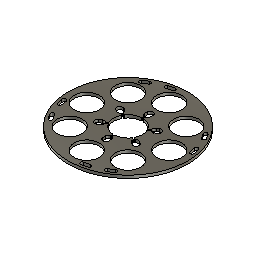
Laser Cut Spool (Autodesk Fusion 360 design; units mm, degrees)
Autodesk Fusion 360 part; units mm, degrees
sketch "Sketch1" plane through (0, 0, 0) normal (0, 0, 1) x (1, 0, 0)
  circle A0 centre (0, 0) radius 100
  circle A1 centre (0, 0) radius 38
  line L0 (0, 0) -> (0, -33) construction
  circle A2 centre (0, -33) radius 5 construction
  circle A3 centre (28.5788, -16.5) radius 5
  circle A4 centre (28.5788, 16.5) radius 5
  circle A5 centre (0, 33) radius 5
  circle A6 centre (-28.5788, 16.5) radius 5
  circle A7 centre (-28.5788, -16.5) radius 5
  circle A8 centre (0, 69) radius 21
  circle A9 centre (0, 0) radius 90
  circle A10 centre (0, 0) radius 48
  line L1 (0, 0) -> (0, 69) construction
  circle A11 centre (0, 0) radius 24
  circle A12 centre (0, 0) radius 28 construction
  line L2 (-0.8255, -28.0686) -> (-0.8255, -23.9858)
  line L3 (0.8255, -23.9858) -> (0.8255, -28.0686)
  line L4 (21.1851, -11.278) -> (24.7209, -13.3194)
  line L5 (23.8954, -14.7492) -> (20.3596, -12.7078)
  line L6 (20.3596, 12.7078) -> (23.8954, 14.7492)
  line L7 (24.7209, 13.3194) -> (21.1851, 11.278)
  line L8 (-0.8255, 23.9858) -> (-0.8255, 28.0686)
  line L9 (0.8255, 28.0686) -> (0.8255, 23.9858)
  line L10 (-21.1851, 11.278) -> (-24.7209, 13.3194)
  line L11 (-23.8954, 14.7492) -> (-20.3596, 12.7078)
  line L12 (-20.3596, -12.7078) -> (-23.8954, -14.7492)
  line L13 (-24.7209, -13.3194) -> (-21.1851, -11.278)
  circle A13 centre (-48.7904, 48.7904) radius 21
  circle A14 centre (-69, 0) radius 21
  circle A15 centre (-48.7904, -48.7904) radius 21
  circle A16 centre (0, -69) radius 21
  circle A17 centre (48.7904, -48.7904) radius 21
  circle A18 centre (69, 0) radius 21
  circle A19 centre (48.7904, 48.7904) radius 21
  arc A20 (-15.8446, 94.6834) -> (-25.6549, 92.5085) centre (0, 0) ccw
  arc A21 (-25.6549, 92.5085) -> (-24.0515, 86.7267) centre (-24.8532, 89.6176) ccw
  arc A22 (-14.8543, 88.7657) -> (-15.8446, 94.6834) centre (-15.3494, 91.7246) ccw
  line L14 (-24.8532, 89.6176) -> (0, 0) construction
  line L15 (-15.3494, 91.7246) -> (0, 0) construction
  line L16 (-20.7782, 93.7244) -> (0, 0) construction
  arc A23 (-44.3181, 78.332) -> (-47.2727, 83.5541) centre (-45.7954, 80.9431) ccw
  arc A24 (-47.2727, 83.5541) -> (-55.7475, 78.1551) centre (0, 0) ccw
  arc A25 (-55.7475, 78.1551) -> (-52.2633, 73.2704) centre (-54.0054, 75.7127) ccw
  arc A26 (-88.7657, -14.8543) -> (-94.6834, -15.8446) centre (-91.7246, -15.3494) ccw
  arc A27 (-92.5085, -25.6549) -> (-86.7267, -24.0515) centre (-89.6176, -24.8532) ccw
  arc A28 (-94.6834, -15.8446) -> (-92.5085, -25.6549) centre (0, 0) ccw
  arc A29 (-83.5541, -47.2727) -> (-78.1551, -55.7475) centre (0, 0) ccw
  arc A30 (-78.1551, -55.7475) -> (-73.2704, -52.2633) centre (-75.7127, -54.0054) ccw
  arc A31 (-78.332, -44.3181) -> (-83.5541, -47.2727) centre (-80.9431, -45.7954) ccw
  arc A32 (14.8543, -88.7657) -> (15.8446, -94.6834) centre (15.3494, -91.7246) ccw
  arc A33 (25.6549, -92.5085) -> (24.0515, -86.7267) centre (24.8532, -89.6176) ccw
  arc A34 (15.8446, -94.6834) -> (25.6549, -92.5085) centre (0, 0) ccw
  arc A35 (47.2727, -83.5541) -> (55.7475, -78.1551) centre (0, 0) ccw
  arc A36 (55.7475, -78.1551) -> (52.2633, -73.2704) centre (54.0054, -75.7127) ccw
  arc A37 (44.3181, -78.332) -> (47.2727, -83.5541) centre (45.7954, -80.9431) ccw
  arc A38 (88.7657, 14.8543) -> (94.6834, 15.8446) centre (91.7246, 15.3494) ccw
  arc A39 (92.5085, 25.6549) -> (86.7267, 24.0515) centre (89.6176, 24.8532) ccw
  arc A40 (94.6834, 15.8446) -> (92.5085, 25.6549) centre (0, 0) ccw
  arc A41 (83.5541, 47.2727) -> (78.1551, 55.7475) centre (0, 0) ccw
  arc A42 (78.1551, 55.7475) -> (73.2704, 52.2633) centre (75.7127, 54.0054) ccw
  arc A43 (78.332, 44.3181) -> (83.5541, 47.2727) centre (80.9431, 45.7954) ccw
  line L17 (-5, -33) -> (-5, -37)
  arc A44 (-5, -37) -> (5, -37) centre (0, -37) ccw
  line L18 (5, -37) -> (5, -33)
  arc A45 (5, -33) -> (-5, -33) centre (0, -33) ccw
  line L19 (0, -33) -> (0, -37) construction
  arc A46 (31.0788, -12.1699) -> (26.0788, -20.8301) centre (28.5788, -16.5) ccw
  line L20 (26.0788, -20.8301) -> (29.5429, -22.8301)
  line L21 (34.5429, -14.1699) -> (31.0788, -12.1699)
  arc A47 (29.5429, -22.8301) -> (34.5429, -14.1699) centre (32.0429, -18.5) ccw
  arc A48 (26.0788, 20.8301) -> (31.0788, 12.1699) centre (28.5788, 16.5) ccw
  line L22 (31.0788, 12.1699) -> (34.5429, 14.1699)
  line L23 (29.5429, 22.8301) -> (26.0788, 20.8301)
  arc A49 (34.5429, 14.1699) -> (29.5429, 22.8301) centre (32.0429, 18.5) ccw
  arc A50 (-5, 33) -> (5, 33) centre (0, 33) ccw
  line L24 (5, 33) -> (5, 37)
  line L25 (-5, 37) -> (-5, 33)
  arc A51 (5, 37) -> (-5, 37) centre (0, 37) ccw
  arc A52 (-31.0788, 12.1699) -> (-26.0788, 20.8301) centre (-28.5788, 16.5) ccw
  line L26 (-26.0788, 20.8301) -> (-29.5429, 22.8301)
  line L27 (-34.5429, 14.1699) -> (-31.0788, 12.1699)
  arc A53 (-29.5429, 22.8301) -> (-34.5429, 14.1699) centre (-32.0429, 18.5) ccw
  arc A54 (-26.0788, -20.8301) -> (-31.0788, -12.1699) centre (-28.5788, -16.5) ccw
  line L28 (-31.0788, -12.1699) -> (-34.5429, -14.1699)
  line L29 (-29.5429, -22.8301) -> (-26.0788, -20.8301)
  arc A55 (-34.5429, -14.1699) -> (-29.5429, -22.8301) centre (-32.0429, -18.5) ccw
  dimension "d1" = 200
  dimension "d5" = 76
  dimension "d6" = 10
  dimension "d9" = 0
  dimension "d10" = 0
  dimension "d12" = 360
  dimension "d13" = -10
  dimension "d14" = 10
  dimension "d18" = 4
  dimension "d20" = 0.8255
  dimension "d22" = 360
  dimension "d23" = 4
  dimension "d25" = 6
  dimension "d29" = 20
  dimension "d30" = 9.5
  dimension "d32" = 360
  dimension "d35" = 4
  dimension "d37" = 360
  constraint concentric A0 A1
  constraint coincident A0.centre A1.centre
  constraint vertical L0
  constraint coincident L0.end A2.centre
  constraint tangent A1 A2
  constraint tangent A8 A10
  constraint tangent A8 A9
  constraint coincident A8.centre L1.end
  constraint concentric A1 A11
  constraint tangent A6 A12
  constraint coincident A11 L2.end
  constraint vertical L2
  constraint coincident A11 L3.start
  constraint coincident A2 L3.end
  constraint parallel L2 L3
  constraint symmetric L0 L2 L3
  constraint concentric A0 A20
  constraint tangent A20 A21
  constraint coincident A9 A21.end
  constraint tangent A9 A21
  constraint tangent A9 A22
  constraint coincident A9 A22.start
  constraint tangent A20 A22
  constraint coincident A21.centre L14.start
  constraint coincident A22.centre L15.start
  constraint midpoint A20 L16.start
  constraint coincident A2 L2.start
  constraint vertical L1
  constraint tangent L17 A44
  constraint tangent A44 L18
  constraint parallel L17 L18
  constraint tangent L18 A45
  constraint tangent L17 A45
  constraint parallel L0 L19
  constraint equal A2 A45
  measures "d1" diameter of A0
  measures "d5" diameter of A1
  measures "d6" diameter of A2
  measures "d20" distance of L0 L3
  measures "d23" distance of A0 A20
  measures "d25" angle of L14 L15
  measures "d30" angle of L1 L15
  measures "d35" distance of L0.end A44.centre
extrude "Extrude1" add sketch "Sketch1" along normal blind 4.7498 contours A0 | A1 A3 A4 A11 L4 L7 A46 L21 A47 A48 L22 A49 | A1 A4 A5 A11 L6 L9 A48 L23 A49 A50 L24 A51 | A1 A3 A11 L3 L5 A44 L18 A45 A46 L20 A47 | A1 A5 A6 A11 L8 L11 A50 L25 A51 A52 L26 A53 | A1 A7 A11 L2 L12 L17 A44 A45 A54 L29 A55 | A1 A6 A7 A11 L10 L13 A52 L27 A53 A54 L28 A55 | A8 A9 A10 A19 | A8 A9 A10 A13 | A10 | A9 A10 A18 A19 | A9 A10 A13 A14 | A9 A10 A17 A18 | A9 A10 A14 A15 | A9 A10 A16 A17 | A9 A10 A15 A16
fillet "Fillet1" radius 1 23 edges at (-20.3596, 12.7078, 2.3749) (-21.1851, 11.278, 2.3749) (-24.7209, 13.3194, 2.3749) (-23.8954, 14.7492, 2.3749) (-0.8255, 23.9858, 2.3749) (-0.8255, 28.0686, 2.3749) (0.8255, 28.0686, 2.3749) (0.8255, 23.9858, 2.3749) (21.1851, 11.278, 2.3749) (24.7209, 13.3194, 2.3749) (23.8954, 14.7492, 2.3749) (20.3596, 12.7078, 2.3749) (23.8954, -14.7492, 2.3749) (24.7209, -13.3194, 2.3749) (21.1851, -11.278, 2.3749) (-20.3596, -12.7078, 2.3749) (-23.8954, -14.7492, 2.3749) (-24.7209, -13.3194, 2.3749) (-21.1851, -11.278, 2.3749) (-0.8255, -23.9858, 2.3749) (0.8255, -23.9858, 2.3749) (-0.8255, -28.0686, 2.3749) (0.8255, -28.0686, 2.3749)
convert_to_sheet_metal "ConvertToSheetMetal1"
sketch "Sketch2" plane through (0, 0, 4.7498) normal (0, 0, 1) x (-1, 0, 0)
  arc A0 (-0.8255, 27.2844) -> (-1.5212, 28.237) centre (-1.8255, 27.2844) ccw
  arc A1 (-5, 33) -> (-1.5212, 28.237) centre (0, 33) ccw
  line L0 (-5, 33) -> (-5, 37)
  arc A2 (5, 37) -> (-5, 37) centre (0, 37) ccw
  line L1 (5, 37) -> (5, 33)
  arc A3 (1.5212, 28.237) -> (5, 33) centre (0, 33) ccw
  arc A4 (1.5212, 28.237) -> (0.8255, 27.2844) centre (1.8255, 27.2844) ccw
  line L2 (0.8255, 27.2844) -> (0.8255, 24.9333)
  arc A5 (0.8255, 24.9333) -> (1.7525, 23.9359) centre (1.8255, 24.9333) ccw
  arc A6 (19.8529, 13.4857) -> (1.7525, 23.9359) centre (0, 0) ccw
  arc A7 (19.8529, 13.4857) -> (21.1801, 13.1815) centre (20.6801, 14.0476) ccw
  line L3 (21.1801, 13.1815) -> (23.2163, 14.3571)
  arc A8 (23.2163, 14.3571) -> (23.6934, 15.436) centre (22.7163, 15.2232) ccw
  arc A9 (26.0788, 20.8301) -> (23.6934, 15.436) centre (28.5788, 16.5) ccw
  line L4 (26.0788, 20.8301) -> (29.5429, 22.8301)
  arc A10 (34.5429, 14.1699) -> (29.5429, 22.8301) centre (32.0429, 18.5) ccw
  line L5 (34.5429, 14.1699) -> (31.0788, 12.1699)
  arc A11 (25.2146, 12.8011) -> (31.0788, 12.1699) centre (28.5788, 16.5) ccw
  arc A12 (25.2146, 12.8011) -> (24.0418, 12.9273) centre (24.5418, 12.0613) ccw
  line L6 (24.0418, 12.9273) -> (22.0056, 11.7517)
  arc A13 (22.0056, 11.7517) -> (21.6054, 10.4503) centre (22.5056, 10.8857) ccw
  arc A14 (21.6054, -10.4503) -> (21.6054, 10.4503) centre (0, 0) ccw
  arc A15 (21.6054, -10.4503) -> (22.0056, -11.7517) centre (22.5056, -10.8857) ccw
  line L7 (22.0056, -11.7517) -> (24.0418, -12.9273)
  arc A16 (24.0418, -12.9273) -> (25.2146, -12.8011) centre (24.5418, -12.0613) ccw
  arc A17 (31.0788, -12.1699) -> (25.2146, -12.8011) centre (28.5788, -16.5) ccw
  line L8 (31.0788, -12.1699) -> (34.5429, -14.1699)
  arc A18 (29.5429, -22.8301) -> (34.5429, -14.1699) centre (32.0429, -18.5) ccw
  line L9 (29.5429, -22.8301) -> (26.0788, -20.8301)
  arc A19 (23.6934, -15.436) -> (26.0788, -20.8301) centre (28.5788, -16.5) ccw
  arc A20 (23.6934, -15.436) -> (23.2163, -14.3571) centre (22.7163, -15.2232) ccw
  line L10 (23.2163, -14.3571) -> (21.1801, -13.1815)
  arc A21 (21.1801, -13.1815) -> (19.8529, -13.4857) centre (20.6801, -14.0476) ccw
  arc A22 (1.7525, -23.9359) -> (19.8529, -13.4857) centre (0, 0) ccw
  arc A23 (1.7525, -23.9359) -> (0.8255, -24.9333) centre (1.8255, -24.9333) ccw
  line L11 (0.8255, -24.9333) -> (0.8255, -27.2844)
  arc A24 (0.8255, -27.2844) -> (1.5212, -28.237) centre (1.8255, -27.2844) ccw
  arc A25 (5, -33) -> (1.5212, -28.237) centre (0, -33) ccw
  line L12 (5, -33) -> (5, -37)
  arc A26 (-5, -37) -> (5, -37) centre (0, -37) ccw
  line L13 (-5, -37) -> (-5, -33)
  arc A27 (-1.5213, -28.237) -> (-5, -33) centre (0, -33) ccw
  arc A28 (-1.5213, -28.237) -> (-0.8255, -27.2844) centre (-1.8255, -27.2844) ccw
  line L14 (-0.8255, -27.2844) -> (-0.8255, -24.9333)
  arc A29 (-0.8255, -24.9333) -> (-1.7525, -23.9359) centre (-1.8255, -24.9333) ccw
  arc A30 (-19.8529, -13.4857) -> (-1.7525, -23.9359) centre (0, 0) ccw
  arc A31 (-19.8529, -13.4857) -> (-21.1801, -13.1815) centre (-20.6801, -14.0476) ccw
  line L15 (-21.1801, -13.1815) -> (-23.2163, -14.3571)
  arc A32 (-23.2163, -14.3571) -> (-23.6934, -15.436) centre (-22.7163, -15.2232) ccw
  arc A33 (-26.0788, -20.8301) -> (-23.6934, -15.436) centre (-28.5788, -16.5) ccw
  line L16 (-26.0788, -20.8301) -> (-29.5429, -22.8301)
  arc A34 (-34.5429, -14.1699) -> (-29.5429, -22.8301) centre (-32.0429, -18.5) ccw
  line L17 (-34.5429, -14.1699) -> (-31.0788, -12.1699)
  arc A35 (-25.2146, -12.8011) -> (-31.0788, -12.1699) centre (-28.5788, -16.5) ccw
  arc A36 (-25.2146, -12.8011) -> (-24.0418, -12.9273) centre (-24.5418, -12.0613) ccw
  line L18 (-24.0418, -12.9273) -> (-22.0056, -11.7517)
  arc A37 (-22.0056, -11.7517) -> (-21.6054, -10.4503) centre (-22.5056, -10.8857) ccw
  arc A38 (-21.6054, 10.4503) -> (-21.6054, -10.4503) centre (0, 0) ccw
  arc A39 (-21.6054, 10.4503) -> (-22.0056, 11.7517) centre (-22.5056, 10.8857) ccw
  line L19 (-22.0056, 11.7517) -> (-24.0418, 12.9273)
  arc A40 (-24.0418, 12.9273) -> (-25.2146, 12.8011) centre (-24.5418, 12.0613) ccw
  arc A41 (-31.0788, 12.1699) -> (-25.2146, 12.8011) centre (-28.5788, 16.5) ccw
  line L20 (-31.0788, 12.1699) -> (-34.5429, 14.1699)
  arc A42 (-29.5429, 22.8301) -> (-34.5429, 14.1699) centre (-32.0429, 18.5) ccw
  line L21 (-29.5429, 22.8301) -> (-26.0788, 20.8301)
  arc A43 (-23.6934, 15.436) -> (-26.0788, 20.8301) centre (-28.5788, 16.5) ccw
  arc A44 (-23.6934, 15.436) -> (-23.2163, 14.3571) centre (-22.7163, 15.2232) ccw
  line L22 (-23.2163, 14.3571) -> (-20.3596, 12.7078)
  arc A45 (-1.7525, 23.9359) -> (-20.3596, 12.7078) centre (0, 0) ccw
  arc A46 (-1.7525, 23.9359) -> (-0.8255, 24.9333) centre (-1.8255, 24.9333) ccw
  line L23 (-0.8255, 24.9333) -> (-0.8255, 27.2844)
  circle A47 centre (0, 69) radius 21
  circle A48 centre (-48.7904, -48.7904) radius 21
  arc A49 (-88.7657, -14.8543) -> (-94.6834, -15.8446) centre (-91.7246, -15.3494) ccw
  arc A50 (-88.7657, -14.8543) -> (-86.7267, -24.0515) centre (0, 0) ccw
  arc A51 (-92.5085, -25.6549) -> (-86.7267, -24.0515) centre (-89.6176, -24.8532) ccw
  arc A52 (-94.6834, -15.8446) -> (-92.5085, -25.6549) centre (0, 0) ccw
  arc A53 (44.3181, -78.332) -> (47.2727, -83.5541) centre (45.7954, -80.9431) ccw
  arc A54 (44.3181, -78.332) -> (52.2633, -73.2704) centre (0, 0) ccw
  arc A55 (55.7475, -78.1551) -> (52.2633, -73.2704) centre (54.0054, -75.7127) ccw
  arc A56 (47.2727, -83.5541) -> (55.7475, -78.1551) centre (0, 0) ccw
  circle A57 centre (-48.7904, 48.7904) radius 21
  arc A58 (-44.3181, 78.332) -> (-47.2727, 83.5541) centre (-45.7954, 80.9431) ccw
  arc A59 (-44.3181, 78.332) -> (-52.2633, 73.2704) centre (0, 0) ccw
  arc A60 (-55.7475, 78.1551) -> (-52.2633, 73.2704) centre (-54.0054, 75.7127) ccw
  arc A61 (-47.2727, 83.5541) -> (-55.7475, 78.1551) centre (0, 0) ccw
  arc A62 (14.8543, -88.7657) -> (15.8446, -94.6834) centre (15.3494, -91.7246) ccw
  arc A63 (14.8543, -88.7657) -> (24.0515, -86.7267) centre (0, 0) ccw
  arc A64 (25.6549, -92.5085) -> (24.0515, -86.7267) centre (24.8532, -89.6176) ccw
  arc A65 (15.8446, -94.6834) -> (25.6549, -92.5085) centre (0, 0) ccw
  arc A66 (-78.332, -44.3181) -> (-83.5541, -47.2727) centre (-80.9431, -45.7954) ccw
  arc A67 (-78.332, -44.3181) -> (-73.2704, -52.2633) centre (0, 0) ccw
  arc A68 (-78.1551, -55.7475) -> (-73.2704, -52.2633) centre (-75.7127, -54.0054) ccw
  arc A69 (-83.5541, -47.2727) -> (-78.1551, -55.7475) centre (0, 0) ccw
  arc A70 (-14.8543, 88.7657) -> (-15.8446, 94.6834) centre (-15.3494, 91.7246) ccw
  arc A71 (-14.8543, 88.7657) -> (-24.0515, 86.7267) centre (0, 0) ccw
  arc A72 (-25.6549, 92.5085) -> (-24.0515, 86.7267) centre (-24.8532, 89.6176) ccw
  arc A73 (-15.8446, 94.6834) -> (-25.6549, 92.5085) centre (0, 0) ccw
  circle A74 centre (-69, 0) radius 21
  arc A75 (78.332, 44.3181) -> (83.5541, 47.2727) centre (80.9431, 45.7954) ccw
  arc A76 (78.332, 44.3181) -> (73.2704, 52.2633) centre (0, 0) ccw
  arc A77 (78.1551, 55.7475) -> (73.2704, 52.2633) centre (75.7127, 54.0054) ccw
  arc A78 (83.5541, 47.2727) -> (78.1551, 55.7475) centre (0, 0) ccw
  circle A79 centre (48.7904, -48.7904) radius 21
  circle A80 centre (48.7904, 48.7904) radius 21
  arc A81 (88.7657, 14.8543) -> (94.6834, 15.8446) centre (91.7246, 15.3494) ccw
  arc A82 (88.7657, 14.8543) -> (86.7267, 24.0515) centre (0, 0) ccw
  arc A83 (92.5085, 25.6549) -> (86.7267, 24.0515) centre (89.6176, 24.8532) ccw
  arc A84 (94.6834, 15.8446) -> (92.5085, 25.6549) centre (0, 0) ccw
  circle A85 centre (0, -69) radius 21
  circle A86 centre (69, 0) radius 21
  circle A87 centre (0, 0) radius 100
equation "d20 = 0.065 in / 2"
